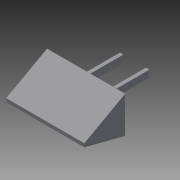
# Autodesk Inventor part: Prow
Saved by Autodesk Inventor 2015 (Build 190159000, 159)
## iProperties
Created: 2016-01-19
Part Number: Prow
Material: Generic
Document SubType Name: Modeling
Designer: sethbattis
Density: 1 g/cm^3
Appearance: Default
Author: sethbattis
Autodesk Inventor part; units mm, degrees
ref_plane "YZ Plane" through (0, 0, 0) normal (1, 0, 0) x (0, 1, 0)
ref_plane "XZ Plane" through (0, 0, 0) normal (0, 1, 0) x (-1, 0, 0)
ref_plane "XY Plane" through (0, 0, 0) normal (0, 0, 1) x (1, 0, 0)
sketch "Sketch1" plane through (0, 0, 0) normal (1, 0, 0) x (0, 1, 0)
  line L0 (-127, -12.7) -> (-127, -77.6639) construction
  line L1 (0, -312.42) -> (0, 496.57) construction
  line L2 (-202.8496, 0) -> (248.9132, 0) construction
  line L3 (76.331, 381) -> (-138.3121, 381) construction
  line L4 (177.8, 0) -> (50.8, 0) construction
  line L5 (50.8, 0) -> (50.8, 50.8) construction
  line L6 (82.55, 82.55) -> (146.05, 82.55) construction
  line L7 (177.8, 50.8) -> (177.8, 0) construction
  arc A0 (177.8, 50.8) -> (146.05, 82.55) centre (146.05, 50.8) ccw construction
  arc A1 (82.55, 82.55) -> (50.8, 50.8) centre (82.55, 50.8) ccw construction
  line L8 (0, 381) -> (-25.4, 381)
  line L9 (-25.4, 381) -> (-102.4194, 82.55)
  line L10 (-102.4194, 82.55) -> (164.7876, 82.55)
  line L11 (164.7876, 82.55) -> (0, 381)
  line L12 (-25.4, 381) -> (-127, -12.7) construction
  line L13 (50.8, -196.85) -> (50.8, 0) construction
  line L14 (50.8, -196.85) -> (0, -196.85) construction
  line L15 (39.8671, 0) -> (0, -196.85) construction
  point P0 (0, 0)
  point P1 (50.8, 82.55)
  point P2 (177.8, 82.55)
  dimension "d2" = 127
  dimension "d3" = 381
  dimension "d4" = 127
  dimension "d5" = 82.55
  dimension "d6" = 304.8
  dimension "d7" = 31.75
  dimension "d8" = 25.4
  dimension "d36" = 196.85
  dimension "d37" = 11.449
  constraints: 28 end point, 11 point on line, 6 tangent, 4 collinear, 4 point on circle, 3 horizontal, 2 centre point, 2 parallel, 2 perpendicular, 1 equal radius, 1 vertical
  measures "d2" distance between parallel lines of L0 L1
  measures "d3" distance between parallel lines of L3 L2
  measures "d4" distance of point (50.8, 82.55) point (177.8, 82.55)
  measures "d5" distance of L4.end point (50.8, 82.55)
  measures "d6" distance between parallel lines of L0 L7
  measures "d7" radius of A0
  measures "d8" distance of L8.start L8.end
  measures "d36" distance of L13.start L13.end
  measures "d37" angle of L1 L15
extrude "Extrusion1" add sketch "Sketch1" along normal blind 571.5
sketch "Sketch2" plane through (0, -102.4194, 82.55) normal (0, 0, -1) x (-1, 0, 0)
  line L0 (0, 0) -> (0, 267.207) construction
  line L1 (0, 267.207) -> (-571.5, 267.207) construction
  line L2 (-571.5, 0) -> (-571.5, 267.207) construction
  line L3 (0, 0) -> (-571.5, 0) construction
  line L4 (-393.7, 153.2194) -> (-368.3, 153.2194)
  line L5 (-368.3, 153.2194) -> (-368.3, 102.4194)
  line L6 (-368.3, 102.4194) -> (-393.7, 102.4194)
  line L7 (-393.7, 102.4194) -> (-393.7, 153.2194)
  line L8 (0, 102.4194) -> (-571.5, 102.4194) projected
  line L9 (-203.2, 153.2194) -> (-177.8, 153.2194)
  line L10 (-177.8, 153.2194) -> (-177.8, 102.4194)
  line L11 (-177.8, 102.4194) -> (-203.2, 102.4194)
  line L12 (-203.2, 102.4194) -> (-203.2, 153.2194)
  line L13 (0, 267.207) -> (-571.5, 267.207) construction
  line L14 (-285.75, 267.207) -> (-285.75, 0) construction
  dimension "d29" = 25.4
  dimension "d30" = 50.8
  dimension "d31" = 215.9
  constraints: 18 end point, 4 parallel, 2 equal length, 2 horizontal, 2 midpoint, 2 perpendicular, 2 point on line, 1 other
  measures "d29" distance of L5.end L6.end
  measures "d30" distance of L4.end L5.end
  measures "d31" distance between parallel lines of L10 L7
extrude "Extrusion2" add sketch "Sketch2" along normal blind 355.6
body "Solid1"
